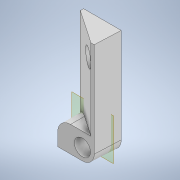
# Autodesk Inventor part: Holder
Saved by Autodesk Inventor 2022 (Build 260153000, 153)
## iProperties
Created: 2021-04-22
Part Number: Holder
Material: Generic
Document SubType Name: Modeling
Designer: Viktor
Density: 1 g/cm^3
Appearance: Default
Author: Viktor
## iProperties of the stored document Holder_3DPrint.ipt
Created: 2021-04-22
Part Number: Holder_3DPrint
Material: Generic
Document SubType Name: Modeling
Designer: Viktor
Density: 1 g/cm^3
Appearance: Default
Author: Viktor
Autodesk Inventor part; units mm, degrees
ref_plane "YZ Plane" through (0, 0, 0) normal (1, 0, 0) x (0, 1, 0)
ref_plane "XZ Plane" through (0, 0, 0) normal (0, 1, 0) x (-1, 0, 0)
ref_plane "XY Plane" through (0, 0, 0) normal (0, 0, 1) x (1, 0, 0)
sketch "Sketch1" plane through (0, 0, 0) normal (0, 0, 1) x (1, 0, 0)
  circle A0 centre (0, 0) radius 12
  line L0 (12, 0) -> (12, 88)
  line L1 (12, 88) -> (-23, 88)
  line L2 (-23, 88) -> (-23, -12)
  line L3 (-23, -12) -> (0, -12)
  dimension "d0" = 24
  dimension "d1" = 100
  dimension "d2" = 35
  constraints: 8 end point, 3 perpendicular, 2 point on circle, 1 centre point, 1 coincident, 1 vertical
  measures "d0" diameter of A0
  measures "d1" distance between parallel lines of L3 L1
  measures "d2" distance between parallel lines of L0 L2
extrude "Extrusion1" add sketch "Sketch1" along normal blind 25
draft "FaceDraft1" angle 2.5 pull direction (0, 0, 1) faces at (-15.3333, -12, 16.6667) (11.866, -1.7885, 16.6667) (12, 29.3333, 16.6667) fixed edges at (-11.5, -12, 0) (8.4853, -8.4853, 0) (12, 44, 0)
sketch "Sketch2" plane through (0, 0, 0) normal (0, 0, -1) x (-1, 0, 0)
  circle A0 centre (0, 0) radius 2.75
  line L0 (0, 0) -> (0, 102) construction
  circle A1 centre (0, 70) radius 2.75
  dimension "d6" = 5.5
  dimension "d16" = 70
  dimension "d17" = 5.5
  constraints: 2 centre point, 2 end point, 1 coincident, 1 point on line, 1 vertical
  measures "d6" diameter of A0
  measures "d16" distance of A1.centre point (0, 0)
  measures "d17" diameter of A1
extrude "Extrusion2" cut sketch "Sketch2" against normal through all
ref_plane "Work Plane1" through (0, 0, 10) normal (0, 0, -1) x (-1, 0, 0)
sketch "Sketch3" plane through (0, 0, 25) normal (0, 0, 1) x (1, 0, 0)
  circle A0 centre (0, 0) radius 2.75 projected
  circle A1 centre (0, 0) radius 7.5
  circle A2 centre (0, 70) radius 2.75 projected
  circle A3 centre (0, 70) radius 2.75 projected
  circle A4 centre (0, 70) radius 7.5
  dimension "d10" = 15
  dimension "d18" = 15
  constraints: 3 coincident, 2 centre point
  measures "d10" diameter of A1
  measures "d18" diameter of A4
extrude "Extrusion3" cut sketch "Sketch3" against normal up to surface (15 mm away)
chamfer "Chamfer1" distance 1 angle 45 7 edges at (8.4853, -8.4853, 0) (12, 44, 0) (-11.5, -12, 0) (2.75, 0, 0) (-5.5, 88, 0) (-23, 38, 0) (2.75, 70, 0)
sketch "Sketch4" plane through (-23, 88, 25) normal (0, 1, 0) x (1, 0, 0)
  line L0 (33.9085, 0) -> (0, 0) projected
  line L1 (0, 24) -> (0, 0) projected
  line L2 (0, 24) -> (0, 21)
  line L3 (0, 24) -> (0, 0) projected
  line L4 (34.9564, 24.001) -> (33.9085, 0) projected
  line L5 (33.9085, 0) -> (30.9085, 0)
  line L6 (23, 0) -> (33.9085, 0) projected
  line L7 (0, 21) -> (30.9085, 0)
  point P0 (30.9085, 0)
  dimension "d20" = 3
  constraints: 6 end point, 2 point on line
  measures "d20" distance of L0.start L5.end
extrude "Extrusion4" cut sketch "Sketch4" against normal blind 75
fillet "Fillet1" radius 12 1 edges at (-23, 13, 14.5)
equation "\"d17\" = d6"
equation "\"d18\" = d10"
body "Solid1"
